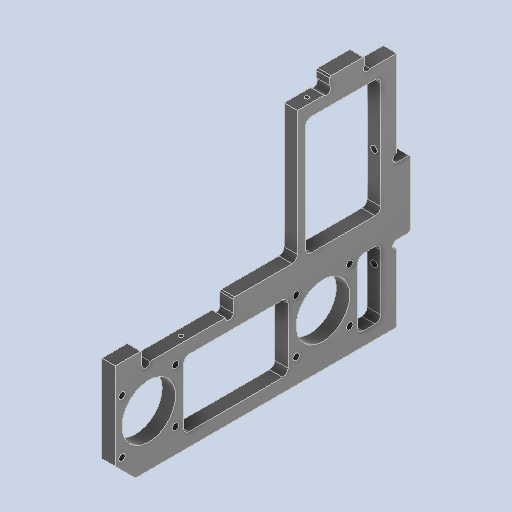
# Autodesk Inventor part: TorsoElectronicBoxSideFrame
Saved by Autodesk Inventor 2024.2 (Build 282272000, 272)
## iProperties
Created: 2024-01-27
Part Number: TorsoElectronicBoxSideFrame
Material: Acetal Resin, Black
Document SubType Name: Modeling
Designer: Masato Kubotera
Density: 1.425 g/cm^3
Appearance: Smooth - Black
Vendor: meviy
Mass: 35.6597 g
Surface Area: 137.332 cm^2
Volume: 25.0244 cm^3
Author: Masato Kubotera
Autodesk Inventor part; units mm, degrees
ref_plane "YZ Plane" through (0, 0, 0) normal (1, 0, 0) x (0, 1, 0)
ref_plane "XZ Plane" through (0, 0, 0) normal (0, 1, 0) x (-1, 0, 0)
ref_plane "XY Plane" through (0, 0, 0) normal (0, 0, 1) x (1, 0, 0)
derived "TorsoSideFrame.ipt"
sketch "Sketch1" plane through (0, 0, 0) normal (0, 1, 0) x (-1, 0, 0)
  circle A0 centre (0, 0) radius 18.75
  line L0 (0, 0) -> (0, -161.5)
  circle A1 centre (0, 0) radius 29 construction
  line L1 (0, 0) -> (0, 36)
  line L2 (0, 36) -> (-48.2759, 36)
  line L3 (-65, -12.5) -> (-65, -118)
  line L4 (-50, -161.5) -> (-35, -161.5)
  line L5 (-35, -161.5) -> (-35, -166.5)
  line L6 (-35, -166.5) -> (-10, -166.5)
  line L7 (-10, -166.5) -> (-10, -161.5)
  line L8 (-10, -161.5) -> (0, -161.5)
  line L9 (-60, -40.225) -> (-65, -40.225)
  line L10 (-44, -161.5) -> (-44, -155.5) construction
  line L11 (-22.5, -166.5) -> (-22.5, -161.5) construction
  arc A2 (-6, -161.5) -> (-10, -161.5) centre (-8, -161.5) ccw
  arc A3 (-35, -161.5) -> (-39, -161.5) centre (-37, -161.5) ccw
  line L12 (-65, -12.5) -> (-60, -12.5) construction
  line L13 (-60, -12.5) -> (-60, -106) construction
  line L14 (-62.5, -12.5) -> (-62.5, -106) construction
  line L15 (-70, -66) -> (0, -66) construction
  line L16 (-65, -40.25) -> (-60, -40.25) construction
  arc A4 (-60, -44.225) -> (-60, -40.225) centre (-60, -42.225) ccw
  line L17 (-60, -111) -> (0, -111) construction
  line L18 (-60, -106) -> (0, -106) construction
  line L19 (-60, -108.5) -> (-17.75, -108.5) construction
  line L20 (-9.95, -111.05) -> (-25.55, -111.05)
  line L21 (-25.55, -111.05) -> (-25.55, -105.95)
  line L22 (-25.55, -105.95) -> (-9.95, -105.95)
  line L23 (-9.95, -105.95) -> (-9.95, -111.05)
  line L24 (-9.95, -111.05) -> (-25.55, -105.95) construction
  line L25 (-25.55, -111.05) -> (-9.95, -105.95) construction
  line L26 (-25.5, -106) -> (-25.5, -111) construction
  arc A5 (-21.55, -105.95) -> (-25.55, -105.95) centre (-23.55, -105.95) ccw
  arc A6 (-25.55, -111.05) -> (-21.55, -111.05) centre (-23.55, -111.05) ccw
  line L27 (-22.5, -76.875) -> (-42.5, -76.875) construction
  line L28 (-42.5, -76.875) -> (-42.5, -96.875) construction
  line L29 (-42.5, -96.875) -> (-22.5, -96.875) construction
  line L30 (-22.5, -96.875) -> (-22.5, -76.875) construction
  line L31 (-22.5, -76.875) -> (-42.5, -96.875) construction
  line L32 (-42.5, -76.875) -> (-22.5, -96.875) construction
  line L33 (-45, -74.375) -> (-20, -74.375)
  line L34 (-20, -74.375) -> (-20, -99.375)
  line L35 (-20, -99.375) -> (-45, -99.375)
  line L36 (-45, -99.375) -> (-45, -74.375)
  line L37 (-45, -74.375) -> (-20, -99.375) construction
  line L38 (-20, -74.375) -> (-45, -99.375) construction
  line L39 (-50, 31) -> (0, 31) construction
  line L40 (-38.05, 31.05) -> (-14.95, 31.05)
  line L41 (-14.95, 31.05) -> (-14.95, 25.95)
  line L42 (-14.95, 25.95) -> (-38.05, 25.95)
  line L43 (-38.05, 25.95) -> (-38.05, 31.05)
  line L44 (-38.05, 31.05) -> (-14.95, 25.95) construction
  line L45 (-14.95, 31.05) -> (-38.05, 25.95) construction
  line L46 (-38.05, 28.5) -> (-14.95, 28.5) construction
  line L47 (-38, 31) -> (-38, 26) construction
  line L48 (-26.5, 31.05) -> (-26.5, 25.95) construction
  line L49 (-15, 31) -> (-15, 26) construction
  arc A7 (-34.05, 31.05) -> (-38.05, 31.05) centre (-36.05, 31.05) ccw
  arc A8 (-38.05, 25.95) -> (-34.05, 25.95) centre (-36.05, 25.95) ccw
  arc A9 (-14.95, 31.05) -> (-18.95, 31.05) centre (-16.95, 31.05) ccw
  arc A10 (-18.95, 25.95) -> (-14.95, 25.95) centre (-16.95, 25.95) ccw
  line L50 (-46.4119, -155.5) -> (-3.5, -155.5)
  arc A11 (-48.3027, -154.152) -> (-46.4119, -155.5) centre (-46.4119, -153.5) ccw
  arc A12 (-3.5, -155.5) -> (-1.5, -153.5) centre (-3.5, -153.5) ccw
  circle A13 centre (-41.25, -65.25) radius 2 construction
  line L51 (-3.5, -62.75) -> (-54, -62.75)
  line L52 (0, 0) -> (-29, 0) construction
  line L53 (-30.7958, -111) -> (-29.7506, -111)
  arc A14 (-27.8427, -112.4) -> (-20.2699, -114.1308) centre (-23.55, -111.05) ccw
  line L54 (-1.5, -153.5) -> (-1.5, -113)
  arc A15 (-1.5, -113) -> (-3.5, -111) centre (-3.5, -113) ccw
  arc A16 (-27.8427, -112.4) -> (-29.7506, -111) centre (-29.7506, -113) ccw
  circle A17 centre (-33.5, -108.5) radius 1.75 construction
  arc A18 (-18.8121, -113.5) -> (-20.2699, -114.1308) centre (-18.8121, -115.5) ccw
  line L55 (-17.75, -105.95) -> (-17.75, -111.05) construction
  arc A19 (-29.7506, -106) -> (-27.8427, -104.6) centre (-29.7506, -104) ccw
  arc A20 (-20.2699, -102.8692) -> (-27.8427, -104.6) centre (-23.55, -105.95) ccw
  arc A21 (-20.2699, -102.8692) -> (-18.8121, -103.5) centre (-18.8121, -101.5) ccw
  line L56 (-10, -106) -> (-10, -111) construction
  arc A22 (-13.95, -111.05) -> (-9.95, -111.05) centre (-11.95, -111.05) ccw
  arc A23 (-5.7494, -111) -> (-7.6573, -112.4) centre (-5.7494, -113) ccw
  arc A24 (-15.2301, -114.1308) -> (-16.6879, -113.5) centre (-16.6879, -115.5) ccw
  arc A25 (-15.2301, -114.1308) -> (-7.6573, -112.4) centre (-11.95, -111.05) ccw
  arc A26 (-9.95, -105.95) -> (-13.95, -105.95) centre (-11.95, -105.95) ccw
  arc A27 (-16.6879, -103.5) -> (-15.2301, -102.8692) centre (-16.6879, -101.5) ccw
  arc A28 (-7.6573, -104.6) -> (-15.2301, -102.8692) centre (-11.95, -105.95) ccw
  arc A29 (-7.6573, -104.6) -> (-5.7494, -106) centre (-5.7494, -104) ccw
  line L57 (-18.8121, -103.5) -> (-16.6879, -103.5)
  line L58 (-18.8121, -113.5) -> (-16.6879, -113.5)
  line L59 (-5.7494, -111) -> (-3.5, -111)
  line L60 (-5.7494, -106) -> (-3.5, -106)
  arc A30 (-3.5, -106) -> (-1.5, -104) centre (-3.5, -104) ccw
  line L61 (-41.25, -65.25) -> (-36.25, -65.25) construction
  line L62 (-60, -44.225) -> (-60, -86.275)
  line L63 (-60, -65.25) -> (-65, -65.25) construction
  line L64 (-65, -90.25) -> (-60, -90.25) construction
  arc A31 (-60, -90.275) -> (-60, -86.275) centre (-60, -88.275) ccw
  line L65 (-60, -90.275) -> (-65, -90.275)
  line L66 (-60, -106) -> (-65, -106) construction
  line L67 (-1.5, -24.2487) -> (-1.5, -60.75)
  line L68 (-54, -67.75) -> (-3.5, -67.75)
  line L69 (-1.5, -69.75) -> (-1.5, -104)
  line L70 (-56, -60.75) -> (-56, -47.5165)
  circle A32 centre (-32.5, -86.875) radius 10
  circle A33 centre (-32.5, -86.875) radius 11
  arc A34 (-15.79, 16.0289) -> (-21.7764, 5.6601) centre (0, 0) ccw
  arc A35 (-21.7764, -5.6601) -> (-15.79, -16.0289) centre (0, 0) ccw
  arc A36 (-5.9864, -21.689) -> (-3.2143, -22.2692) centre (0, 0) ccw
  arc A37 (-24.0442, 4.191) -> (-24.0442, -4.191) centre (-24.75, 0) ccw
  line L71 (-48.2759, 36) -> (-65, -12.5)
  arc A38 (-42.9869, 36) -> (-50, 31) centre (-42.9869, 28.5817) ccw
  line L72 (-75.1102, 42.6949) -> (-93.0397, -9.3006) construction
  ellipse E0 centre (-84.0749, 16.6972) end of major axis (-76.7401, 37.9681) minor radius 15 construction
  ellipse E1 centre (-84.0749, 16.6972) end of major axis (-93.0397, -9.3006) minor radius 20 construction
  line L73 (-75.1102, 42.6949) -> (-76.7401, 37.9681) construction
  line L74 (-105, 43.5) -> (-105, 11.4504) construction
  line L75 (-84.0749, 16.6972) -> (-58.029, 7.7158) construction
  line L76 (-63.4041, 25.9649) -> (-39.2683, 17.6422) construction
  line L77 (-39.2683, 17.6422) -> (-49.374, -11.6643) construction
  line L78 (-49.374, -11.6643) -> (-73.5098, -3.3416) construction
  line L79 (-79.9787, 43.5) -> (-105, 43.5) construction
  line L80 (-47.0676, 20.3317) -> (-57.1733, -8.9749) construction
  circle A39 centre (-49.757, 12.5323) radius 6.25 construction
  circle A40 centre (-54.4839, -1.1756) radius 6.25 construction
  line L81 (-1, 13.5) -> (-28, 13.5) construction
  line L82 (-28, 13.5) -> (-28, -13.5) construction
  line L83 (-28, -13.5) -> (-1, -13.5) construction
  line L84 (-1, -13.5) -> (-1, 13.5) construction
  line L85 (-1, 13.5) -> (-28, -13.5) construction
  line L86 (-28, 13.5) -> (-1, -13.5) construction
  line L87 (0, -65.25) -> (-64.9996, -65.25) construction
  line L88 (-50, -161.5) -> (-65, -118)
  line L89 (-18.3182, 21.5) -> (-45.3395, 21.5)
  arc A41 (-16.4164, 20.1189) -> (-15.6516, 18.7274) centre (-12.375, 21.4341) ccw
  arc A42 (-55.5, -46.1936) -> (-58.5, -36.4155) centre (-60, -42.225) ccw
  arc A43 (-48.7278, 6.3677) -> (-46.4104, 17.8109) centre (-49.757, 12.5323) ccw
  arc A44 (-48.7278, 6.3677) -> (-49.8737, 3.0445) centre (-48.3985, 4.395) ccw
  arc A45 (-56.6994, -7.0197) -> (-49.8737, 3.0445) centre (-54.4839, -1.1756) ccw
  line L90 (-38, 26) -> (-15, 26) construction
  line L91 (-59.2992, -8.2378) -> (-59.8907, -9.9535)
  line L92 (-48.3027, -154.152) -> (-49.1959, -151.5616)
  arc A46 (-47.8996, -149) -> (-48.7278, -136.8677) centre (-49.757, -143.0323) ccw
  arc A47 (-49.8737, -133.5445) -> (-48.7278, -136.8677) centre (-48.3985, -134.895) ccw
  arc A48 (-49.8737, -133.5445) -> (-56.6994, -123.4803) centre (-54.4839, -129.3244) ccw
  line L93 (-59.2992, -122.2622) -> (-59.8907, -120.5465)
  line L94 (-60, -119.8946) -> (-60, -113)
  circle A49 centre (-41.25, -65.25) radius 1 construction
  line L95 (-45, -86.875) -> (-20, -86.875) construction
  arc A50 (-45.3395, 21.5) -> (-46.4104, 17.8109) centre (-45.3395, 19.5) ccw
  arc A51 (-56.6994, -7.0197) -> (-59.2992, -8.2378) centre (-57.4084, -8.8898) ccw
  arc A52 (-16.4164, 20.1189) -> (-18.3182, 21.5) centre (-18.3182, 19.5) ccw
  arc A53 (-15.79, 16.0289) -> (-15.6516, 18.7274) centre (-17.1936, 17.4537) ccw
  arc A54 (-24.0442, 4.191) -> (-21.7764, 5.6601) centre (-23.7121, 6.1632) ccw
  arc A55 (-21.7764, -5.6601) -> (-24.0442, -4.191) centre (-23.7121, -6.1632) ccw
  arc A56 (-15.6516, -18.7274) -> (-15.79, -16.0289) centre (-17.1936, -17.4537) ccw
  arc A57 (-5.9864, -21.689) -> (-8.3926, -22.9184) centre (-6.5186, -23.6169) ccw
  arc A58 (-60, -34.479) -> (-58.5, -36.4155) centre (-58, -34.479) ccw
  line L96 (-40, -42.225) -> (-60, -42.225) construction
  circle A59 centre (-33.5, -108.5) radius 3.25 construction
  arc A60 (-35.174, -111.2857) -> (-31.826, -111.2857) centre (-33.5, -108.5) ccw
  line L97 (-36.2042, -111) -> (-58, -111)
  line L98 (-36.2042, -106) -> (-58, -106)
  arc A61 (-31.826, -105.7143) -> (-35.174, -105.7143) centre (-33.5, -108.5) ccw
  line L99 (-30.7958, -106) -> (-29.7506, -106)
  arc A62 (-58.5, -94.0845) -> (-55.5, -84.3064) centre (-60, -88.275) ccw
  arc A63 (-58.5, -94.0845) -> (-60, -96.021) centre (-58, -96.021) ccw
  line L100 (-56, -69.75) -> (-56, -82.9835)
  line L101 (-60, -96.021) -> (-60, -104)
  arc A64 (-36.2042, -106) -> (-35.174, -105.7143) centre (-36.2042, -104) ccw
  arc A65 (-35.174, -111.2857) -> (-36.2042, -111) centre (-36.2042, -113) ccw
  arc A66 (-60, -104) -> (-58, -106) centre (-58, -104) ccw
  arc A67 (-58, -111) -> (-60, -113) centre (-58, -113) ccw
  circle A68 centre (-36.25, -65.25) radius 2 construction
  arc A69 (-31.826, -105.7143) -> (-30.7958, -106) centre (-30.7958, -104) ccw
  arc A70 (-30.7958, -111) -> (-31.826, -111.2857) centre (-30.7958, -113) ccw
  arc A71 (-47.8996, -149) -> (-49.1959, -151.5616) centre (-47.3052, -150.9096) ccw
  arc A72 (-59.2992, -122.2622) -> (-56.6994, -123.4803) centre (-57.4084, -121.6102) ccw
  arc A73 (-60, -119.8946) -> (-59.8907, -120.5465) centre (-58, -119.8946) ccw
  arc A74 (-60, -119.8946) -> (-59.8907, -120.5465) centre (-58, -119.8946) ccw
  arc A75 (-56, -82.9835) -> (-55.5, -84.3064) centre (-54, -82.9835) ccw
  arc A76 (-54, -67.75) -> (-56, -69.75) centre (-54, -69.75) ccw
  arc A77 (-56, -60.75) -> (-54, -62.75) centre (-54, -60.75) ccw
  arc A78 (-55.5, -46.1936) -> (-56, -47.5165) centre (-54, -47.5165) ccw
  arc A79 (-1.5, -69.75) -> (-3.5, -67.75) centre (-3.5, -69.75) ccw
  arc A80 (-3.5, -62.75) -> (-1.5, -60.75) centre (-3.5, -60.75) ccw
  line L102 (-18.3182, -21.5) -> (-58, -21.5)
  arc A81 (-18.3182, -21.5) -> (-16.4164, -20.1189) centre (-18.3182, -19.5) ccw
  arc A82 (-15.6516, -18.7274) -> (-16.4164, -20.1189) centre (-12.375, -21.4341) ccw
  arc A83 (-14.5, -25.1147) -> (-8.3926, -22.9184) centre (-12.375, -21.4341) ccw
  line L103 (-16.0857, -24.5) -> (-58, -24.5)
  arc A84 (-1.5, -24.2487) -> (-3.2143, -22.2692) centre (-3.5, -24.2487) ccw
  line L104 (-60, -10.6054) -> (-60, -19.5)
  line L105 (-60, -26.5) -> (-60, -34.479)
  arc A85 (-59.8907, -9.9535) -> (-60, -10.6054) centre (-58, -10.6054) ccw
  arc A86 (-60, -19.5) -> (-58, -21.5) centre (-58, -19.5) ccw
  arc A87 (-58, -24.5) -> (-60, -26.5) centre (-58, -26.5) ccw
  arc A88 (-15.0479, -24.7903) -> (-14.5, -25.1147) centre (0, 0) ccw
  arc A89 (-15.0479, -24.7903) -> (-16.0857, -24.5) centre (-16.0857, -26.5) ccw
  point P0 (-16.05, -9.6933)
  point P1 (-12.375, -21.4341)
  point P2 (12.375, -21.4341)
  point P3 (24.75, 0)
  point P4 (12.375, 21.4341)
  point P5 (-70, -66)
  point P6 (0, -66)
  point P7 (-47.5, -132.5)
  point P8 (-26.5, 28.5)
  point P9 (-60, -106)
  point P10 (-46, 28.5)
  point P11 (-56, -62.75)
  point P12 (-1.5, -155.5)
  point P13 (-5, -161.5)
  point P14 (-28.0497, -111)
  point P15 (-28.0239, -110.5665)
  point P16 (-1.5, -62.75)
  point P17 (-7.4503, -111)
  point P18 (-56, -67.75)
  point P19 (-1.5, -67.75)
  point P20 (-1.5, -22.4499)
  point P21 (-38, 28.5)
  point P22 (-14.5, 0)
  point P23 (-1, 0)
  point P24 (-16.6245, 21.5)
  point P25 (-56, -46.6971)
  point P26 (-60, -36.225)
  point P27 (-49.9833, 18.7782)
  point P28 (-58.5118, -5.9545)
  point P29 (-60, -10.2703)
  point P30 (-46.2796, -23.3529)
  point P31 (-31.2796, -23.3529)
  point P32 (-46.2796, -46.6256)
  point P33 (-62.5, -30.25)
  point P34 (-62.5, -100.25)
  point P35 (-49.9833, -149.2782)
  point P36 (-58.5118, -124.5455)
  point P37 (-60, -120.2297)
  point P38 (-36.05, 23.95)
  point P39 (-31.4233, -111)
  point P40 (-31.4233, -106)
  point P41 (-56, -83.8029)
  point P42 (-40, -88.275)
  point P43 (-15.5161, -24.5)
sketch "Sketch2" plane through (0, 0, 0) normal (0, 1, 0) x (-1, 0, 0)
  arc A0 (60, -77.75) -> (60, -80.75) centre (60, -79.25) ccw
  line L0 (60, -83.75) -> (54, -83.75) construction
  line L1 (65, -77.75) -> (60, -77.75)
  line L2 (60, -77.75) -> (60, -106)
  line L3 (60, -46.75) -> (54, -46.75) construction
  line L4 (60, -12.5) -> (60, -52.75)
  line L5 (65, -65.25) -> (60, -65.25) construction
  line L6 (60, -52.75) -> (65, -52.75)
  line L7 (65, -52.75) -> (65, -77.75)
  arc A1 (60, -49.75) -> (60, -52.75) centre (60, -51.25) ccw
  line L8 (60, -106) -> (-45, -106)
  line L9 (-45, -106) -> (-45, -66)
  line L10 (23, -66) -> (23, -12.5)
  line L11 (23, -12.5) -> (60, -12.5)
  line L12 (23, -17.5) -> (35, -17.5)
  line L13 (35, -17.5) -> (35, -12.5)
  line L14 (48, -12.5) -> (48, -17.5)
  line L15 (48, -17.5) -> (60, -17.5)
  line L16 (41.5, -12.5) -> (41.5, -17.5) construction
  arc A2 (32.8787, -17.5) -> (35, -15.3787) centre (33.9393, -16.4393) ccw
  line L17 (29, -17.5) -> (29, -23.5) construction
  arc A3 (48, -15.3787) -> (50.1213, -17.5) centre (49.0607, -16.4393) ccw
  line L18 (-35, -66) -> (-1, -66) construction
  line L19 (-1, -66) -> (-1, -71) construction
  line L20 (-1, -71) -> (-35, -71) construction
  line L21 (-35, -71) -> (-35, -66) construction
  line L22 (-35, -66) -> (-1, -71) construction
  line L23 (-1, -66) -> (-35, -71) construction
  line L24 (-35, -68.5) -> (-1, -68.5) construction
  line L25 (-18, -66) -> (-18, -71) construction
  line L26 (-0.95, -71) -> (-35.05, -71)
  line L27 (-35.05, -71) -> (-35.05, -66)
  line L28 (-0.95, -66) -> (-0.95, -71)
  arc A4 (-35.05, -71) -> (-32.05, -71) centre (-33.55, -71) ccw
  arc A5 (-3.95, -71) -> (-0.95, -71) centre (-2.45, -71) ccw
  line L29 (-60, -12.5) -> (-60, -106) construction
  line L30 (0, 0) -> (0, -161.5) construction
  line L31 (60, -12.5) -> (60, -106) construction
  line L32 (-70, -66) -> (0, -66) construction
  line L33 (-60, -106) -> (0, -106) construction
  line L34 (-65, -12.5) -> (-60, -12.5) construction
  line L35 (26, -22) -> (26, -66)
  line L36 (26, -66) -> (54, -66)
  line L37 (54, -66) -> (54, -22)
  line L38 (54, -22) -> (26, -22)
  line L39 (-45, -66) -> (-35.05, -66)
  line L40 (23, -66) -> (-0.95, -66)
  line L41 (45.5, -76) -> (54, -76)
  line L42 (54, -76) -> (54, -101)
  line L43 (54, -101) -> (45.5, -101)
  line L44 (45.5, -101) -> (45.5, -76)
  circle A6 centre (-32.5, -86.875) radius 10 projected
  circle A7 centre (32.5, -86.875) radius 10
  line L45 (-19.5, -76) -> (19.5, -76)
  line L46 (19.5, -76) -> (19.5, -101)
  line L47 (19.5, -101) -> (-19.5, -101)
  line L48 (-19.5, -101) -> (-19.5, -76)
  circle A8 centre (-22.5, -76.875) radius 3 construction
  circle A9 centre (42.5, -76.875) radius 3 construction
  point P0 (-18, -68.5)
  point P1 (-41, -68.5)
  point P2 (5, -68.5)
  point P3 (-42.5, -76.875)
  point P4 (-42.5, -96.875)
  point P5 (-22.5, -96.875)
  point P6 (42.5, -96.875)
  point P7 (22.5, -96.875)
  point P8 (22.5, -76.875)
  point P9 (-0.95, -71)
  point P10 (-3.95, -71)
  point P11 (-30.05, -61.55)
  point P12 (-30.05, -61.55)
  point P13 (50.1213, -17.5)
  point P14 (48, -15.3787)
  point P15 (-0.95, -71)
  dimension "d1" = 25
  dimension "d2" = 6
  dimension "d3" = 1.5
  dimension "d5" = 6
  dimension "d7" = 5
  dimension "d8" = 6
  dimension "d9" = 6
  dimension "d11" = 5
  dimension "d13" = 0.05
  dimension "d15" = 6
  dimension "d19" = 25
  dimension "d20" = 15
  dimension "d21" = 35
  dimension "d22" = 5
  dimension "d23" = 34
  dimension "d24" = 37
  dimension "d64" = 3
  dimension "d65" = 12
  dimension "d68" = 4.5
  dimension "d69" = 93.5
  dimension "d71" = 52.75
  dimension "d80" = 5
  dimension "d81" = 5
  dimension "d82" = 6
  constraints: 88 end point, 18 symmetric about line, 16 point on line, 14 horizontal, 13 point on circle, 11 collinear, 9 centre point, 9 midpoint, 8 vertical, 6 parallel, 6 perpendicular, 3 equal radius, 3 tangent, 2 coincident, 8 other
  measures "d1" distance of L7.start L7.end
  measures "d2" distance of L3.start L3.end
  measures "d3" radius of A1
  measures "d5" distance between parallel lines of L3 L6
  measures "d7" distance between parallel lines of L12 L11
  measures "d8" distance of L17.start L17.end
  measures "d9" distance between parallel lines of L13 L17
  measures "d11" distance of L18.end L20.start
  measures "d13" distance between parallel lines of L27 L21
  measures "d15" distance from line of point (-41, -68.5) L21
  measures "d19" distance between parallel lines of L21 L29
  measures "d20" distance between parallel lines of L29 L9
  measures "d21" distance between parallel lines of L8 L20
  measures "d22" distance of L7.end L2.start
  measures "d23" distance between parallel lines of L21 L19
  measures "d24" distance of L11.start L4.start
  measures "d64" distance between parallel lines of L10 L35
  measures "d65" distance between parallel lines of L10 L13
  measures "d68" distance between parallel lines of L38 L12
  measures "d69" distance between parallel lines of L8 L11
  measures "d71" vertical distance of L5.start L4.start
  measures "d80" distance between parallel lines of L45 L20
  measures "d81" distance between parallel lines of L33 L47
  measures "d82" diameter of A8
extrude "Extrusion1" add sketch "Sketch2" against normal blind 5 contours A0 L2 L8 L9 L39 L27 A4 L26 A5 L28 L40 L10 L12 A2 L13 L11 L14 A3 L15 L4 A1 L6 L7 L1
hole "M3" at (42.5, 0, -76.875) at (42.5, 0, -96.875) at (22.5, 0, -96.875) at (22.5, 0, -76.875) at (-22.5, 0, -76.875) at (-22.5, 0, -96.875) at (-42.5, 0, -96.875) at (-42.5, 0, -76.875) direction (0, -1, 0) diameter 2.459 end through all thread size "M3x0.5" class "6H" standard "ANSI Metric M Profile"
sketch "Sketch3" plane through (-60, 0, -49.75) normal (-1, 0, 0) x (0, 0, -1)
  line L0 (3, 5) -> (0, 5) projected
  line L1 (-3, 5) -> (-3, 0)
  line L2 (28, 5) -> (56.25, 5) projected
  line L3 (34, 5) -> (34, 0)
  point P0 (-49.75, 0)
  point P1 (-32.25, 5)
  point P2 (31, 5)
  point P3 (-3, 0)
  point P4 (-3, 0)
  point P5 (-3, 0)
  point P6 (34, 0)
  point P7 (34, 0)
  point P8 (34, 0)
  point P9 (-3, 2.5)
  point P10 (34, 2.5)
  point P11 (-49.25, 5)
  constraints: 4 end point, 2 coincident, 2 midpoint, 2 point on line, 2 vertical
hole "Side-M3" at (-60, -2.5, -46.75) at (-60, -2.5, -83.75) direction (1, 0, 0) diameter 2.459 depth 6 thread size "M3x0.5" class "6H" standard "ANSI Metric M Profile"
sketch "Sketch4" plane through (-32.8787, 0, -17.5) normal (0, 0, 1) x (-1, 0, 0)
  line L0 (-9.8787, 5) -> (0, 5) projected
  line L1 (-3.8787, 5) -> (-3.8787, 0)
  point P0 (-32.8787, 0)
  point P1 (-3.8787, 0)
  point P2 (-3.8787, 0)
  point P3 (-3.8787, 0)
  point P4 (-3.8787, 2.5)
  constraints: 2 end point, 1 coincident, 1 midpoint, 1 point on line, 1 vertical
hole "Top-M3" at (-29, -2.5, -17.5) direction (0, 0, -1) diameter 1.567 depth 6 thread size "M2x0.4" class "6H" standard "ANSI Metric M Profile"
sketch "Sketch5" plane through (3.95, 0, -71) normal (0, 0, 1) x (1, 0, 0)
  line L0 (14.05, -5) -> (14.05, 0)
  line L1 (0, 0) -> (28.1, 0) projected
  line L2 (28.1, -5) -> (0, -5) projected
  point P0 (-3.95, 0)
  point P1 (14.05, -2.5)
  constraints: 3 midpoint, 2 end point
hole "Top-M2" at (18, -2.5, -71) direction (0, 0, -1) diameter 1.567 depth 6 thread size "M2x0.4" class "6H" standard "ANSI Metric M Profile"
fillet "R2" radius 2 13 edges at (-23, -2.5, -66) (-26, -2.5, -66) (-26, -2.5, -22) (-54, -2.5, -22) (-54, -2.5, -66) (19.5, -2.5, -76) (-19.5, -2.5, -76) (-19.5, -2.5, -101) (19.5, -2.5, -101) (-45.5, -2.5, -76) (-54, -2.5, -76) (-45.5, -2.5, -101) (-54, -2.5, -101)
chamfer "C0.5" distance 0.5 angle 45 6 edges at (-48, -2.5, -12.5) (-35, -2.5, -12.5) (-65, -2.5, -52.75) (-65, -2.5, -77.75) (35.05, -2.5, -66) (0.95, -2.5, -66)
chamfer "C7.5" distance 7.5 angle 45 1 edges at (45, -2.5, -106)
equation "\"d49\" = d2"
body "Solid1"
